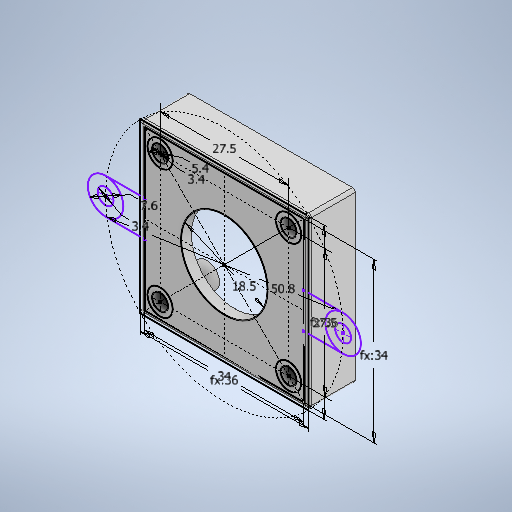
# Autodesk Inventor part: cameraTop
Saved by Autodesk Inventor 2025 (Build 290162000, 162)
## iProperties
Created: 2025-03-10
Part Number: cameraTop
Material: Generic
Document SubType Name: Modeling
Designer: john
Density: 1 g/cm^3
Appearance: Default
Author: john
Autodesk Inventor part; units mm, degrees
ref_plane "YZ Plane" through (0, 0, 0) normal (1, 0, 0) x (0, 1, 0)
ref_plane "XZ Plane" through (0, 0, 0) normal (0, 1, 0) x (-1, 0, 0)
ref_plane "XY Plane" through (0, 0, 0) normal (0, 0, 1) x (1, 0, 0)
sketch "Sketch1" plane through (0, 0, 0) normal (0, 0, 1) x (1, 0, 0)
  circle A0 centre (0, 0) radius 25.4 construction
  line L0 (-13.75, -13.75) -> (13.75, -13.75) construction
  line L1 (13.75, -13.75) -> (13.75, 13.75) construction
  line L2 (13.75, 13.75) -> (-13.75, 13.75) construction
  line L3 (-13.75, 13.75) -> (-13.75, -13.75) construction
  line L4 (-13.75, -13.75) -> (13.75, 13.75) construction
  line L5 (13.75, -13.75) -> (-13.75, 13.75) construction
  circle A1 centre (0, 0) radius 9.25
  circle A2 centre (-13.75, 13.75) radius 1.7
  circle A3 centre (-13.75, 13.75) radius 2.7
  circle A4 centre (-25.4, 0) radius 1.7
  circle A5 centre (-25.4, 0) radius 3.8
  line L6 (-17, 17) -> (17, 17)
  line L7 (17, 17) -> (17, -17)
  line L8 (17, -17) -> (-17, -17)
  line L9 (-17, -17) -> (-17, 17)
  line L10 (-17, 17) -> (17, -17) construction
  line L11 (17, 17) -> (-17, -17) construction
  line L12 (-25.4, 3.8) -> (-18, 3.8)
  line L13 (-25.4, -3.8) -> (-18, -3.8)
  line L14 (0, 17) -> (0, -17) construction
  line L15 (-17, 0) -> (17, 0) construction
  circle A6 centre (25.4, 0) radius 1.7
  circle A7 centre (25.4, 0) radius 3.8
  line L16 (25.4, 3.8) -> (18, 3.8)
  line L17 (25.4, -3.8) -> (18, -3.8)
  circle A8 centre (13.75, 13.75) radius 1.7
  circle A9 centre (13.75, 13.75) radius 2.7
  circle A10 centre (-13.75, -13.75) radius 1.7
  circle A11 centre (-13.75, -13.75) radius 2.7
  circle A12 centre (13.75, -13.75) radius 2.7
  circle A13 centre (13.75, -13.75) radius 1.7
  line L18 (-18, 18) -> (18, 18)
  line L19 (18, 18) -> (18, -18)
  line L20 (18, -18) -> (-18, -18)
  line L21 (-18, -18) -> (-18, 18)
  line L22 (-18, 18) -> (18, -18) construction
  line L23 (18, 18) -> (-18, -18) construction
  point P0 (-17, 3.8)
  point P1 (-17, -3.8)
  point P2 (17, 3.8)
  point P3 (17, -3.8)
  dimension "d0" = 50.8
  dimension "d1" = 27.5
  dimension "d2" = 27.5
  dimension "d3" = 18.5
  dimension "d4" = 3.4
  dimension "d5" = 5.4
  dimension "d6" = 3.4
  dimension "d7" = 7.6
  dimension "d8" = 34
  dimension "d9" = 34
  dimension "d10" = 36
  dimension "d11" = 36
  constraints: 48 end point, 17 coincident, 14 centre point, 12 symmetric about line, 10 midpoint, 6 parallel, 6 point on circle, 6 point on line, 5 perpendicular, 3 horizontal, 2 tangent, 8 other
  measures "d0" diameter of A0
  measures "d1" distance of L2.end L1.end
  measures "d2" distance of L1.end L0.end
  measures "d3" diameter of A1
  measures "d4" diameter of A2
  measures "d5" diameter of A3
  measures "d6" diameter of A4
  measures "d7" diameter of A5
  measures "d8" distance of L7.end L8.end
  measures "d9" distance of L6.end L7.end
  measures "d10" distance of L19.end L20.end
  measures "d11" distance of L18.end L19.end
extrude "Extrusion1" add sketch "Sketch1" against normal blind 10 contours A3 | L21 L18 L19 L20 | A9 | A11 | A12
extrude "Extrusion2" add sketch "Sketch1" against normal blind 2.2 contours L6 L7 L8 L9
fillet "Fillet1" radius 0.6 8 edges at (18, 0, 0) (0, 18, 0) (-18, 0, 0) (0, -18, 0) (18, 18, -5) (-18, 18, -5) (-18, -18, -5) (18, -18, -5)
equation "\"d9\" = d8"
body "Solid1"
